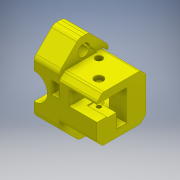
# Autodesk Inventor part: Y Carriage 1.0
Saved by Autodesk Inventor 2016 (Build 200138000, 138)
## iProperties
Created: 2017-01-26
Part Number: Y Carriage 1.0
Material: PET Plastic
Document SubType Name: Modeling
Designer: Scott
Density: 1.541 g/cm^3
Appearance: Smooth - Yellow
Author: Scott
## iProperties of the stored document Y Carriage 1.0_3DPrint.ipt
Created: 2017-04-10
Part Number: Y Carriage 1.0_3DPrint
Material: Generic
Document SubType Name: Modeling
Designer: Scott
Density: 1 g/cm^3
Appearance: Default
Author: Scott
Autodesk Inventor part; units mm, degrees
ref_plane "YZ Plane" through (0, 0, 0) normal (1, 0, 0) x (0, 1, 0)
ref_plane "XZ Plane" through (0, 0, 0) normal (0, 1, 0) x (-1, 0, 0)
sketch "Sketch1" plane through (0, 0, 0) normal (0, 0, 1) x (1, 0, 0)
  line L0 (0, 17.5) -> (45, 17.5)
  line L1 (45, 17.5) -> (45, -17.5)
  line L2 (45, -17.5) -> (0, -17.5)
  line L3 (0, -17.5) -> (0, 17.5)
  point P0 (0, 0)
  dimension "d0" = 35
  dimension "d1" = 45
  dimension "d2" = 17.5
  constraints: 8 end point, 2 parallel, 1 horizontal, 1 midpoint, 1 perpendicular
  measures "d0" distance between parallel lines of L2 L0
  measures "d1" distance of L0.start L0.end
  measures "d2" distance from line of point (0, 0) L0
sketch "Sketch1 outline for Extrusion1" plane through (0, 0, 0) normal (0, 0, 1) x (1, 0, 0)
  line L0 (0, 17.5) -> (45, 17.5)
  line L1 (45, 17.5) -> (45, -17.5)
  line L2 (45, -17.5) -> (0, -17.5)
  line L3 (0, -17.5) -> (0, 17.5)
extrude "Extrusion1" add sketch "Sketch1 outline for Extrusion1" along normal mid plane 33
sketch "Sketch2" plane through (0, 0, 16.5) normal (0, 0, 1) x (1, 0, 0)
  point P0 (0, 0)
  point P1 (22.5, 6.365)
  point P2 (35.23, -6.365)
  dimension "d5" = 6.365
  dimension "d6" = 6.365
  dimension "d7" = 22.5
  dimension "d8" = 12.73
  measures "d5" vertical distance of point (0, 0) point (22.5, 6.365)
  measures "d6" vertical distance of point (0, 0) point (35.23, -6.365)
  measures "d7" horizontal distance of point (0, 0) point (22.5, 6.365)
  measures "d8" horizontal distance of point (35.23, -6.365) point (22.5, 6.365)
hole "Hole1" at (22.5, 6.365, 16.5) at (35.23, -6.365, 16.5) direction (0, 0, -1) diameter 3 end through all
sketch "Sketch3" plane through (0, 0, 0) normal (0, 0, 1) x (1, 0, 0)
  circle A0 centre (35.23, -6.365) radius 1.5
  arc A1 (35.23, 3.635) -> (25.23, -6.365) centre (35.23, -6.365) ccw
  line L0 (0, -17.5) -> (45, -17.5)
  line L1 (45, -17.5) -> (45, 17.5)
  line L2 (45, 17.5) -> (45, -17.5)
  line L3 (35.23, -6.365) -> (35.23, 6.603315) construction
  line L4 (35.23, -6.365) -> (21.82885, -6.365) construction
  line L5 (35.23, 3.635) -> (45, 3.635)
  line L6 (25.23, -6.365) -> (25.23, -17.5)
  line L7 (45, -17.5) -> (0, -17.5)
  line L8 (25.23, -17.5) -> (45, -17.5)
  line L9 (45, -17.5) -> (45, 3.635)
  point P0 (0, 0)
  dimension "d16" = 20
  constraints: 12 end point, 4 perpendicular, 4 point on line, 2 point on circle, 1 centre point, 1 coincident, 1 horizontal, 1 tangent, 1 vertical
  measures "d16" diameter of A1
sketch "Sketch3 outline for Extrusion2" plane through (0, 0, 0) normal (0, 0, 1) x (1, 0, 0)
  line L0 (25.23, -17.5) -> (45, -17.5)
  line L1 (25.23, -6.365) -> (25.23, -17.5)
  line L2 (45, -17.5) -> (45, 3.635)
  arc A0 (35.23, 3.635) -> (25.23, -6.365) centre (35.23, -6.365) ccw
  line L3 (45, 3.635) -> (35.23, 3.635)
  circle A1 centre (35.23, -6.365) radius 1.5
extrude "Extrusion2" cut sketch "Sketch3 outline for Extrusion2" along normal blind 11
sketch "Sketch4" plane through (0, 0, 0) normal (0, 0, 1) x (1, 0, 0)
  circle A0 centre (22.5, 6.365) radius 1.5
  arc A1 (12.5, 6.365) -> (22.5, -3.635) centre (22.5, 6.365) ccw
  line L0 (45, 17.5) -> (0, 17.5)
  line L1 (45, -17.5) -> (45, 17.5)
  line L2 (22.5, 6.365) -> (6.341938, 6.365) construction
  line L3 (22.5, 6.365) -> (22.5, -7.410166) construction
  line L4 (12.5, 6.365) -> (12.5, 17.5)
  line L5 (0, 17.5) -> (45, 17.5) construction
  line L6 (22.5, -3.635) -> (45, -3.635)
  line L7 (45, 3.635) -> (35.23, 3.635)
  line L8 (45, 3.635) -> (45, -17.5)
  line L9 (45, 3.635) -> (32.5, 3.635)
  line L10 (32.5, 3.635) -> (32.5, 17.5)
  line L11 (12.5, 17.5) -> (32.5, 17.5)
  line L12 (45, 3.635) -> (45, -3.635)
  point P0 (0, 0)
  dimension "d19" = 20
  dimension "d20" = 10
  constraints: 16 end point, 6 point on line, 2 collinear, 2 perpendicular, 2 point on circle, 2 vertical, 1 centre point, 1 coincident, 1 horizontal, 1 tangent
  measures "d19" diameter of A1
  measures "d20" distance from line of A0.centre L10
sketch "Sketch4 outline for Extrusion3" plane through (0, 0, 0) normal (0, 0, 1) x (1, 0, 0)
  line L0 (22.5, -3.635) -> (45, -3.635)
  arc A0 (12.5, 6.365) -> (22.5, -3.635) centre (22.5, 6.365) ccw
  line L1 (12.5, 17.5) -> (12.5, 6.365)
  line L2 (32.5, 17.5) -> (12.5, 17.5)
  line L3 (32.5, 3.635) -> (32.5, 17.5)
  line L4 (45, 3.635) -> (32.5, 3.635)
  line L5 (45, -3.635) -> (45, 3.635)
extrude "Extrusion3" cut sketch "Sketch4 outline for Extrusion3" against normal blind 11
sketch "Sketch5" plane through (0, -17.5, 16.5) normal (0, -1, 0) x (1, 0, 0)
  line L0 (25.23, -5.5) -> (45, -5.5)
  line L1 (22.5, -16.5) -> (12.5, -16.5)
  line L2 (18, -15.5) -> (18, -6.5)
  line L3 (12.5, -6.5) -> (12.5, -15.5)
  line L4 (18, -15.5) -> (12.5, -15.5)
  line L5 (32.5, -16.5) -> (12.5, -16.5) construction
  line L6 (12.5, -16.5) -> (12.5, 9.231563) construction
  line L7 (12.5, -6.5) -> (18, -6.5)
  point P0 (0, -16.5)
  dimension "d24" = 5.5
  dimension "d27" = 1
  dimension "d28" = 5.5
  dimension "d29" = 25.73156
  dimension "d59" = 1
  constraints: 10 end point, 2 perpendicular, 2 point on line, 1 parallel, 1 vertical
  measures "d24" distance of L2.end L3.start
  measures "d27" distance between parallel lines of L4 L1
  measures "d28" distance between parallel lines of L6 L2
  measures "d29" distance from line of L6.end L5
  measures "d59" distance between parallel lines of L0 L7
sketch "Sketch5 outline for Extrusion4" plane through (0, -17.5, 16.5) normal (0, -1, 0) x (1, 0, 0)
  line L0 (12.5, -15.5) -> (18, -15.5)
  line L1 (12.5, -6.5) -> (12.5, -15.5)
  line L2 (18, -6.5) -> (12.5, -6.5)
  line L3 (18, -15.5) -> (18, -6.5)
extrude "Extrusion4" cut sketch "Sketch5 outline for Extrusion4" against normal through all
sketch "Sketch7" plane through (0, 0, 11) normal (0, 0, -1) x (-1, 0, 0)
  circle A0 centre (-35.23, -6.365) radius 1.5 projected
  circle A1 centre (-35.23, -6.365) radius 2.75
  point P0 (0, 0)
  dimension "d33" = 5.5
  constraints: 1 centre point, 1 coincident
  measures "d33" diameter of A1
sketch "Sketch7 outline for Extrusion6" plane through (0, 0, 11) normal (0, 0, -1) x (-1, 0, 0)
  circle A0 centre (-35.23, -6.365) radius 2.75
extrude "Extrusion6" add sketch "Sketch7 outline for Extrusion6" along normal blind 0.8 draft -30
sketch "Sketch8" plane through (0, 0, 16.5) normal (0, 0, 1) x (1, 0, 0)
  circle A0 centre (35.23, -6.365) radius 1.5 projected
  point P0 (0, 0)
  constraints: 1 coincident
hole "Hole2" at (35.23, -6.365, 16.5) direction (0, 0, -1) diameter 3 end through all counterbore diameter 6.2 counterbore depth 3
sketch "Sketch9" plane through (0, 0, -11) normal (0, 0, 1) x (1, 0, 0)
  circle A0 centre (22.5, 6.365) radius 1.5 projected
  circle A1 centre (22.5, 6.365) radius 2.75
  point P0 (0, 0)
  dimension "d43" = 5.5
  constraints: 1 centre point, 1 coincident
  measures "d43" diameter of A1
sketch "Sketch9 outline for Extrusion7" plane through (0, 0, -11) normal (0, 0, 1) x (1, 0, 0)
  circle A0 centre (22.5, 6.365) radius 2.75
extrude "Extrusion7" add sketch "Sketch9 outline for Extrusion7" along normal blind 0.8 draft -30
sketch "Sketch10" plane through (0, 0, 0) normal (0, 0, -1) x (-1, 0, 0)
  circle A0 centre (-22.5, 6.365) radius 1.5 projected
  circle A1 centre (-22.5, 6.365) radius 2.75
  point P0 (0, 0)
  dimension "d46" = 5.5
  constraints: 1 centre point, 1 coincident
  measures "d46" diameter of A1
sketch "Sketch10 outline for Extrusion8" plane through (0, 0, 0) normal (0, 0, -1) x (-1, 0, 0)
  circle A0 centre (-22.5, 6.365) radius 2.75
extrude "Extrusion8" add sketch "Sketch10 outline for Extrusion8" along normal blind 0.8 draft -30
sketch "Sketch11" plane through (0, 0, -16.5) normal (0, 0, -1) x (-1, 0, 0)
  circle A0 centre (-22.5, 6.365) radius 1.5
  circle A1 centre (-22.5, 6.365) radius 2.28812
  point P0 (0, 0)
  constraints: 1 coincident
hole "Hole3" at (22.5, 6.365, -16.5) direction (0, 0, 1) diameter 3 end through all counterbore diameter 6.2 counterbore depth 3
sketch "Sketch12" plane through (0, 0, 0) normal (0, 1, 0) x (-1, 0, 0)
  circle A0 centre (0, 0) radius 9.5
  dimension "d56" = 19
  constraints: 1 centre point, 1 coincident
  measures "d56" diameter of A0
sketch "Sketch12 outline for Extrusion9" plane through (0, 0, 0) normal (0, 1, 0) x (-1, 0, 0)
  circle A0 centre (0, 0) radius 9.5
extrude "Extrusion9" cut sketch "Sketch12 outline for Extrusion9" along normal through all both and the other way through all
sketch "Sketch13" plane through (0, -17.5, 16.5) normal (-1, 0, 0) x (0, 0, 1)
  line L0 (-16.5, 17.5) -> (25.414559, 17.5) construction
  circle A0 centre (6, 17.5) radius 4.2
  line L1 (-7, 35) -> (0, 35)
  line L2 (-33, 35) -> (-26, 35)
  line L3 (-26, 0) -> (-33, 0)
  line L4 (0, 0) -> (-7, 0)
  line L5 (0, 35) -> (0, 0)
  line L6 (-33, 0) -> (-33, 35)
  line L7 (0, 0) -> (0, 35)
  line L8 (0, 35) -> (1, 35)
  line L9 (1, 35) -> (15, 21)
  line L10 (15, 21) -> (15, 14)
  line L11 (15, 14) -> (1, 0)
  line L12 (1, 0) -> (0, 0)
  dimension "d60" = 8.4
  dimension "d62" = 22.5
  dimension "d64" = 31.5
  dimension "d65" = 1
  dimension "d66" = 1
  dimension "d67" = 45
  dimension "d68" = 45
  constraints: 12 end point, 2 horizontal, 1 centre point, 1 parallel, 1 perpendicular, 1 point on line
  measures "d60" diameter of A0
  measures "d62" distance of A0.centre L0.start
  measures "d64" distance from line of L0.start L10
  measures "d65" distance of L1.end L8.end
  measures "d66" distance of L11.end L4.start
  measures "d67" angle of L5 L9
  measures "d68" angle of L5 L11
sketch "Sketch13 outline for Extrusion10" plane through (0, -17.5, 16.5) normal (-1, 0, 0) x (0, 0, 1)
  line L0 (1, 35) -> (0, 35)
  line L1 (15, 21) -> (1, 35)
  line L2 (0, 35) -> (0, 0)
  line L3 (15, 14) -> (15, 21)
  line L4 (0, 0) -> (1, 0)
  line L5 (1, 0) -> (15, 14)
  circle A0 centre (6, 17.5) radius 4.2
extrude "Extrusion10" add sketch "Sketch13 outline for Extrusion10" against normal blind 18
mirror "Mirror1" about plane through (0, 0, 0) normal (0, 0, 1) of "Extrusion10"
chamfer "Chamfer1" distance 4 angle 45 4 edges at (31.5, -17.5, 16.5) (31.5, 17.5, 16.5) (31.5, -17.5, -16.5) (31.5, 17.5, -16.5)
fillet "Fillet1" radius 5 8 edges at (9, -3.5, 31.5) (9, 3.5, 31.5) (9, 17.5, 17.5) (9, -17.5, 17.5) (9, -17.5, -17.5) (9, -3.5, -31.5) (9, 3.5, -31.5) (9, 17.5, -17.5)
fillet "Fillet2" radius 2 8 edges at (31.5, 13.5, 16.5) (31.5, -13.5, 16.5) (31.5, 17.5, 12.5) (31.5, 17.5, -12.5) (31.5, -17.5, 12.5) (31.5, -17.5, -12.5) (31.5, 13.5, -16.5) (31.5, -13.5, -16.5)
sketch "Sketch14" plane through (0, 0, 16.5) normal (0, 0, 1) x (1, 0, 0)
  circle A0 centre (22.5, 6.365) radius 1.5 projected
  point P0 (0, 0)
  constraints: 1 coincident
hole "Hole4" at (22.5, 6.365, 16.5) direction (0, 0, -1) diameter 4.5 depth 5 counterbore diameter 5 counterbore depth 0.5
sketch "Sketch15" plane through (0, 0, -16.5) normal (0, 0, -1) x (-1, 0, 0)
  circle A0 centre (-35.23, -6.365) radius 1.5 projected
  circle A1 centre (-35.23, -6.365) radius 1.5 projected
  point P0 (0, 0)
  constraints: 1 coincident
hole "Hole5" at (35.23, -6.365, -16.5) direction (0, 0, 1) diameter 4.5 depth 5 counterbore diameter 5 counterbore depth 0.5
sketch "Sketch16" plane through (45, -17.5, 11) normal (1, 0, 0) x (0, 0, -1)
  line L0 (22, 13.865) -> (11, 13.865) projected
  line L1 (11, 13.865) -> (11, 0) projected
  line L2 (11, 13.865) -> (11.8, 13.865)
  line L3 (11.8, 13.865) -> (11.8, 7.05)
  line L4 (11.8, 7.05) -> (11, 7.05)
  line L5 (11, 7.05) -> (11, 13.865)
  point P0 (11, 17.5)
  dimension "d94" = 0.8
  dimension "d95" = 7.05
  constraints: 8 end point, 2 parallel, 1 horizontal, 1 perpendicular
  measures "d94" distance between parallel lines of L1 L3
  measures "d95" distance from line of L1.end L4
sketch "Sketch16 outline for Extrusion11" plane through (45, -17.5, 11) normal (1, 0, 0) x (0, 0, -1)
  line L0 (11, 13.865) -> (11.8, 13.865)
  line L1 (11.8, 13.865) -> (11.8, 7.05)
  line L2 (11.8, 7.05) -> (11, 7.05)
  line L3 (11, 7.05) -> (11, 13.865)
extrude "Extrusion11" cut sketch "Sketch16 outline for Extrusion11" against normal blind 14
fillet "Fillet7" radius 0.2 2 edges at (38, -3.635, -0.8) (38, -10.45, 0)
sketch "Sketch17" plane through (0, -17.5, 9.5) normal (-1, 0, 0) x (0, 0, 1)
  line L0 (-9.5, 17.5) -> (-9.5, -18.967834) construction
  line L1 (-9.5, 17.5) -> (29.523244, 17.5) construction
  line L2 (3, 30) -> (-22, 30) construction
  line L3 (-22, 30) -> (-22, 5) construction
  line L4 (-22, 5) -> (3, 5) construction
  line L5 (3, 5) -> (3, 30) construction
  point P0 (3, 17.5)
  point P1 (-9.5, 5)
  dimension "d99" = 25
  dimension "d100" = 25
  constraints: 12 end point, 4 coincident, 2 horizontal, 2 midpoint, 2 parallel, 2 point on line, 1 perpendicular, 1 vertical
  measures "d99" distance of L3.end L4.end
  measures "d100" distance of L4.end L2.start
hole "Hole6" at (0, 12.5, 12.5) at (0, 12.5, -12.5) at (0, -12.5, -12.5) at (0, -12.5, 12.5) direction (1, 0, 0) diameter 3.2 depth 10 tip angle 118
hole "Hole7" at (0, 12.5, 12.5) at (0, -12.5, 12.5) at (0, -12.5, -12.5) at (0, 12.5, -12.5) direction (1, 0, 0) diameter 4.7 depth 5 counterbore diameter 5 counterbore depth 0.5
sketch "Sketch20" plane through (0, 16.035534, 18.964466) normal (0, 0.7071068, 0.7071068) x (1, 0, 0)
  line L0 (0, 0) -> (18, 0)
  line L1 (0, -15.656854) -> (0, 0)
  line L2 (18, -15.656854) -> (0, -15.656854)
  line L3 (18, 0) -> (18, -15.656854)
  line L4 (-9, -13.838835) -> (54, -13.838835)
  line L5 (18, -15.656854) -> (0, -15.656854) construction
  point P0 (0, 2.071068)
  point P1 (6, -6.338835)
  dimension "d128" = 7.5
  dimension "d129" = 6
  measures "d128" distance from line of point (6, -6.339) L4
  measures "d129" distance from line of point (6, -6.339) L1
hole "Hole9" at (6, 11.553301, 23.446699) direction (0, -0.7071068, -0.7071068) diameter 3.5 depth 30 tip angle 118 counterbore diameter 6 counterbore depth 3
ref_plane "Work Plane1" through (0, 5.428932, 8.357864) normal (0, 0.7071068, 0.7071068) x (1, 0, 0)
sketch "Sketch21" plane through (0, 5.428932, 8.357864) normal (0, 0.7071068, 0.7071068) x (1, 0, 0)
  line L0 (6, -2.374733) -> (9, -4.106784)
  line L1 (9, -4.106784) -> (9, -7.570886)
  line L2 (9, -7.570886) -> (6, -9.302936)
  line L3 (6, -9.302936) -> (3, -7.570886)
  line L4 (3, -7.570886) -> (3, -4.106784)
  line L5 (3, -4.106784) -> (6, -2.374733)
  point P0 (0, 2.071068)
  point P1 (6, -5.838835)
  point P2 (6, -5.838835)
  dimension "d138" = 6
  constraints: 12 end point, 1 coincident, 1 vertical, 13 other
  measures "d138" distance between parallel lines of L1 L4
sketch "Sketch21 outline for Extrusion13" plane through (0, 5.428932, 8.357864) normal (0, 0.7071068, 0.7071068) x (1, 0, 0)
  line L0 (6, -2.374733) -> (9, -4.106784)
  line L1 (9, -4.106784) -> (9, -7.570886)
  line L2 (9, -7.570886) -> (6, -9.302936)
  line L3 (6, -9.302936) -> (3, -7.570886)
  line L4 (3, -7.570886) -> (3, -4.106784)
  line L5 (3, -4.106784) -> (6, -2.374733)
extrude "Extrusion13" cut sketch "Sketch21 outline for Extrusion13" against normal blind 15
sketch "Sketch22" plane through (18, -17.5, 16.5) normal (1, 0, 0) x (0, 0, -1)
  line L0 (0, 4.828427) -> (0, 30.171573)
  arc A0 (0.585786, 31.585786) -> (0, 30.171573) centre (2, 30.171573) ccw
  line L1 (0.585786, 31.585786) -> (3.414214, 34.414214)
  circle A1 centre (-6, 17.5) radius 4.2
  line L2 (-6, 17.5) -> (17.034225, 40.534225) construction
  arc A2 (-2.464466, 1.464466) -> (1.071068, 0) centre (1.071068, 5) ccw
  line L3 (1.071068, 0) -> (4.828427, 0)
  arc A3 (3.414214, 0.585786) -> (4.828427, 0) centre (4.828427, 2) ccw
  line L4 (0.585786, 3.414214) -> (3.414214, 0.585786)
  arc A4 (0, 4.828427) -> (0.585786, 3.414214) centre (2, 4.828427) ccw
  line L5 (0, 30.171573) -> (0, 4.828427)
  arc A5 (0.585786, 31.585786) -> (0, 30.171573) centre (2, 30.171573) ccw
  line L6 (3.414214, 34.414214) -> (0.585786, 31.585786)
  arc A6 (4.828427, 35) -> (3.414214, 34.414214) centre (4.828427, 33) ccw
  line L7 (4.828427, 35) -> (1.071068, 35)
  arc A7 (1.071068, 35) -> (-2.464466, 33.535534) centre (1.071068, 30) ccw
  line L8 (-2.464466, 33.535534) -> (-13.535534, 22.464466)
  arc A8 (-13.535534, 22.464466) -> (-15, 18.928932) centre (-10, 18.928932) ccw
  line L9 (-15, 18.928932) -> (-15, 16.071068)
  arc A9 (-15, 16.071068) -> (-13.535534, 12.535534) centre (-10, 16.071068) ccw
  line L10 (-13.535534, 12.535534) -> (-2.464466, 1.464466)
  circle A10 centre (-6, 17.5) radius 4.2
  line L11 (-5.381347, 21.654187) -> (0, 27.035534)
  line L12 (4.897339, 19.684136) -> (-3.587942, 28.169417)
  line L13 (2.93934, 35) -> (0.055456, 32.116117)
  arc A11 (0.055456, 32.116117) -> (-0.75, 30.171573) centre (2, 30.171573) ccw
  line L14 (-0.75, 30.171573) -> (-0.75, 27.346194)
  line L15 (-6.41694, 21.679254) -> (-0.75, 27.346194)
  point P0 (16.5, 17.5)
  dimension "d141" = 2.5
  dimension "d144" = 0.75
  dimension "d145" = 0.75
  dimension "d146" = 0.75
  dimension "d147" = 2.75
  constraints: 10 end point, 4 point on circle, 3 parallel, 2 point on line, 1 centre point, 1 perpendicular
  measures "d141" distance between parallel lines of L11 L2
  measures "d144" distance between parallel lines of L11 L15
  measures "d145" distance between parallel lines of L0 L14
  measures "d146" distance between parallel lines of L1 L13
  measures "d147" radius of A11
sketch "Sketch22 outline for Extrusion14" plane through (18, -17.5, 16.5) normal (1, 0, 0) x (0, 0, -1)
  line L0 (0, 27.035534) -> (0, 30.171573)
  line L1 (-5.381347, 21.654187) -> (0, 27.035534)
  arc A0 (-6.41694, 21.679254) -> (-5.381347, 21.654187) centre (-6, 17.5) cw
  line L2 (-0.75, 27.346194) -> (-6.41694, 21.679254)
  line L3 (-0.75, 30.171573) -> (-0.75, 27.346194)
  arc A1 (0.055456, 32.116117) -> (-0.75, 30.171573) centre (2, 30.171573) ccw
  line L4 (2.93934, 35) -> (0.055456, 32.116117)
  line L5 (4.828427, 35) -> (2.93934, 35)
  arc A2 (3.414214, 34.414214) -> (4.828427, 35) centre (4.828427, 33) cw
  line L6 (0.585786, 31.585786) -> (3.414214, 34.414214)
  arc A3 (0, 30.171573) -> (0.585786, 31.585786) centre (2, 30.171573) cw
extrude "Extrusion14" cut sketch "Sketch22 outline for Extrusion14" against normal through all
fillet "Fillet8" radius 0.5 3 edges at (9, 4.1793, 22.9169) (9, 4.1542, 21.8813) (9, 17.5, 13.5607)
mirror "Mirror3" about plane through (0, 0, 0) normal (0, 0, 1) of "Extrusion13", "Extrusion14", "Hole9"
equation "\"d2\" = 0.5 * d0"
equation "\"d6\" = d5"
body "Solid1"
